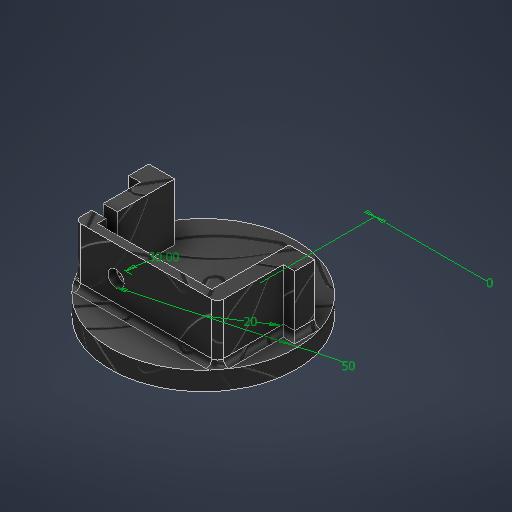
# Autodesk Inventor part: rotacniZaklad
Saved by Autodesk Inventor 2026 (Build 300175000, 175)
## iProperties
Created: 2025-04-11
Part Number: rotacniZaklad
Material: Generic
Document SubType Name: Modeling
Designer: vitgr
Density: 1 g/cm^3
Appearance: Diamond plate 2 - Dark Gray
Author: vitgr
Autodesk Inventor part; units mm, degrees
ref_plane "YZ Plane" through (0, 0, 0) normal (1, 0, 0) x (0, 1, 0)
ref_plane "XZ Plane" through (0, 0, 0) normal (0, 1, 0) x (-1, 0, 0)
ref_plane "XY Plane" through (0, 0, 0) normal (0, 0, 1) x (1, 0, 0)
sketch "Sketch1" plane through (0, 0, 0) normal (0, 1, 0) x (-1, 0, 0)
  line L0 (17.3205, -10) -> (21.6506, -12.5)
  line L1 (0, 0) -> (25, 0) construction
  line L2 (17.3205, 10) -> (21.6506, 12.5)
  line L3 (-17.3205, -10) -> (-21.6506, -12.5)
  line L4 (-17.3205, 10) -> (-21.6506, 12.5)
  arc A0 (17.3205, 10) -> (-17.3205, 10) centre (0, 0) ccw
  arc A1 (-17.3205, -10) -> (17.3205, -10) centre (0, 0) ccw
  arc A2 (21.6506, 12.5) -> (-21.6506, 12.5) centre (0, 0) ccw
  arc A3 (-21.6506, -12.5) -> (21.6506, -12.5) centre (0, 0) ccw
  circle A4 centre (0, 0) radius 25
  point P0 (0, -20)
  point P1 (0, -20)
  dimension "d13" = 50
  dimension "d4" = 30
  dimension "d10" = 0
  dimension "d11" = 20
  constraints: 10 end point, 10 point on circle, 4 centre point, 2 coincident, 1 horizontal, 1 symmetric about line, 3 other
  measures "d4" angle of L0 L1
  measures "d10" distance of point (0, -20) point (0, -20)
  measures "d11" radius of A1
sketch "Sketch2" plane through (0, 0, 0) normal (0, 1, 0) x (-1, 0, 0)
  circle A0 centre (0, 0) radius 32.5
  dimension "d14" = 65
  constraints: 1 centre point, 1 coincident
  measures "d14" diameter of A0
extrude "Extrusion1" add sketch "Sketch2" along normal blind 6.5
sketch "Sketch11" plane through (0, 6.5, 0) normal (0, 1, 0) x (1, 0, 0)
  line L0 (25, 10) -> (20, 10)
  line L1 (20, 10) -> (20, -20)
  line L2 (20, -20) -> (25, -20)
  line L3 (25, -20) -> (25, 10)
  line L4 (25, -20) -> (-25, -20)
  line L5 (-25, -20) -> (-25, -17.0323)
  line L6 (-25, -17.0323) -> (25, -17.0323)
  line L7 (25, -17.0323) -> (25, -20)
  line L8 (-25, -20) -> (-20, -20)
  line L9 (-20, -20) -> (-20, 10)
  line L10 (-20, 10) -> (-25, 10)
  line L11 (-25, 10) -> (-25, -20)
  circle A0 centre (0, 0) radius 32.5 projected
  line L12 (20, 10) -> (29, 10)
  line L13 (29, 10) -> (29, 3)
  line L14 (29, 3) -> (20, 3)
  line L15 (20, 3) -> (20, 10)
  line L16 (0, 45) -> (0, 40)
  line L17 (-25, 10) -> (-20, 10)
  line L18 (-20, 10) -> (-20, -20)
  line L19 (-25, -20) -> (-25, 10)
  line L20 (-20, 10) -> (-29, 10)
  line L21 (-29, 10) -> (-29, 3)
  line L22 (-29, 3) -> (-20, 3)
  line L23 (-20, 3) -> (-20, 10)
  point P0 (0, -20)
  point P1 (20, -17.0323)
  point P2 (-20, -17.0323)
  point P3 (-25, 3)
  point P4 (25, 3)
  dimension "d79" = 30
  dimension "d80" = 50
  dimension "d81" = 5
  dimension "d82" = 5
  dimension "d83" = 30
  dimension "d85" = 25
  dimension "d86" = 25
  dimension "d87" = 20
  dimension "d90" = 9
  dimension "d91" = 7
  dimension "d92" = 9
  dimension "d118" = 40
  constraints: 48 end point, 8 parallel, 4 horizontal, 4 perpendicular, 3 symmetric about line, 1 midpoint, 1 vertical
  measures "d79" distance of L8.end L9.end
  measures "d80" distance of L2.end L4.end
  measures "d81" distance of L0.start L0.end
  measures "d82" distance of L9.end L10.end
  measures "d83" distance of L0.end L1.end
  measures "d85" distance from line of L3 point (0, 0)
  measures "d86" distance from line of point (0, 0) L11
  measures "d87" distance of point (0, 0) point (0, -20)
  measures "d90" distance of L13.end L14.end
  measures "d91" distance of L12.end L13.end
  measures "d92" distance of L9.end L21.start
  measures "d118" distance between parallel lines of L9 L1
extrude "Extrusion9" add sketch "Sketch11" along normal blind 20 contours L3 L14 L1 L0 | L12 L13 L14 L3 | L3 L6 L1 L14 | L3 L2 L1 L6 | L1 L4 L9 L6 | L9 L4 L5 L6 | L6 L11 L22 L9 | L22 L11 L10 L9 | L22 L21 L20 L11
sketch "Sketch12" plane through (-20, 6.5, -10) normal (0, 0, -1) x (-1, 0, 0)
  circle A0 centre (4, 5) radius 1.5
  line L0 (-14, -36) -> (-14, -31)
  line L1 (-14, -31) -> (-21, -31)
  circle A1 centre (4, 15) radius 1.5
  circle A2 centre (-44, 5) radius 1.5
  circle A3 centre (-44, 15) radius 1.5
  line L2 (9, 0) -> (9, 20) projected
  line L3 (12.5, 0) -> (-52.5, 0) projected
  point P0 (-20, -6.5)
  dimension "d93" = 3
  dimension "d96" = 10
  dimension "d99" = 48
  dimension "d102" = 5
  dimension "d103" = 5
  constraints: 4 centre point, 4 end point, 2 vertical, 1 horizontal, 6 other
  measures "d93" diameter of A0
  measures "d96" distance of A0.centre A1.centre
  measures "d99" distance of A0.centre A2.centre
  measures "d102" distance from line of L2 A0.centre
  measures "d103" distance from line of L3 A0.centre
extrude "Extrusion10" cut sketch "Sketch12" against normal blind 5.2
sketch "Sketch13" plane through (-25, 6.5, -3) normal (-1, 0, 0) x (0, 0, 1)
  line L0 (13, 1) -> (17, 1)
  line L1 (17, 1) -> (17, 51)
  line L2 (17, 51) -> (13, 51)
  line L3 (13, 51) -> (13, 1)
  line L4 (35.5, 0) -> (-29.5, 0) projected
  line L5 (23, 0) -> (23, 20) projected
  point P0 (3, -6.5)
  dimension "d108" = 50
  dimension "d109" = 1
  dimension "d110" = 6
  dimension "d111" = 4
  constraints: 8 end point, 2 parallel, 1 horizontal, 1 perpendicular
  measures "d108" distance of L2.end L0.start
  measures "d109" distance between parallel lines of L4 L0
  measures "d110" distance between parallel lines of L1 L5
  measures "d111" distance of L0.start L0.end
extrude "Extrusion11" cut sketch "Sketch13" against normal blind 5.2
fillet "Fillet3" radius 2 9 edges at (-25, 16.5, 20) (25, 16.5, 20) (0, 6.5, 20) (25, 6.5, 8.5) (-25, 6.5, 8.5) (-29, 6.5, -6.5) (-27, 6.5, -3) (29, 6.5, -6.5) (27, 6.5, -3)
sketch "Sketch14" plane through (-23, 26.5, 20) normal (0, 0, 1) x (1, 0, 0)
  circle A0 centre (12.5, -10.5) radius 2.825
  line L0 (3, -20) -> (3, 0) projected
  line L1 (46, -18) -> (0, -18) projected
  point P0 (23, -26.5)
  dimension "d113" = 5.65
  dimension "d114" = 9.5
  dimension "d115" = 7.5
  constraints: 1 centre point
  measures "d113" diameter of A0
  measures "d114" distance from line of L0 A0.centre
  measures "d115" distance from line of L1 A0.centre
extrude "Extrusion12" cut sketch "Sketch14" against normal blind 10
sketch "Sketch15" plane through (0, 0, 0) normal (0, -1, 0) x (1, 0, 0)
  circle A0 centre (6.5, 0) radius 1.3
  circle A1 centre (14.6, 0) radius 1.3
  circle A2 centre (0, 6.5) radius 1.3
  circle A3 centre (0, 14.6) radius 1.3
  circle A4 centre (-6.5, 0) radius 1.3
  circle A5 centre (-14.6, 0) radius 1.3
  circle A6 centre (0, -6.5) radius 1.3
  circle A7 centre (0, -14.6) radius 1.3
  point P0 (0, 0)
  dimension "d119" = 2.6
  dimension "d120" = 2.6
  dimension "d121" = 6.5
  dimension "d122" = 8.1
  dimension "d125" = 360
  constraints: 8 centre point, 17 other
  measures "d119" diameter of A0
  measures "d120" diameter of A1
  measures "d121" distance of A0.centre point (0, 0)
  measures "d122" distance of A1.centre A0.centre
extrude "Extrusion13" cut sketch "Sketch15" against normal blind 4
body "Solid1"
